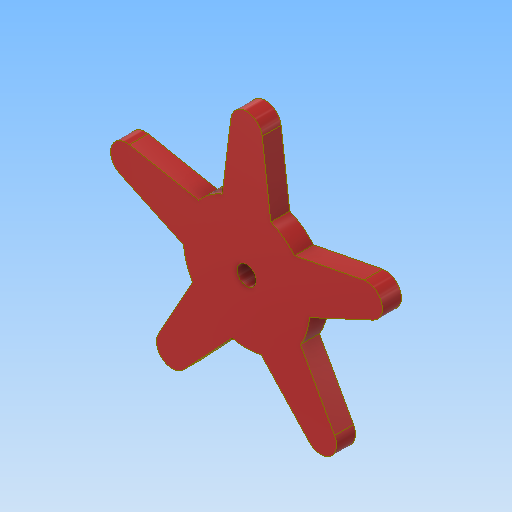
# Autodesk Inventor part: Selection_Gear 1
Saved by Autodesk Inventor 2018.1 (Build 221171000, 171)
## iProperties
Created: 2019-02-16
Part Number: Selection_Gear 1
Material: Nylon 6/6
Document SubType Name: Modeling
Designer: James
Density: 1.13 g/cm^3
Appearance: Nylon 6
Mass: 2.30103 g
Surface Area: 18.9934 cm^2
Volume: 2.03631 cm^3
Author: James
Autodesk Inventor part; units mm, degrees
ref_plane "YZ Plane" through (0, 0, 0) normal (1, 0, 0) x (0, 1, 0)
ref_plane "XZ Plane" through (0, 0, 0) normal (0, 1, 0) x (-1, 0, 0)
ref_plane "XY Plane" through (0, 0, 0) normal (0, 0, 1) x (1, 0, 0)
sketch "Sketch1" plane through (0, 0, 0) normal (0, 0, 1) x (1, 0, 0)
  circle A0 centre (0, 0) radius 10
  dimension "d0" = 20
  constraints: 1 centre point, 1 coincident
  measures "d0" diameter of A0
extrude "Extrusion1" add sketch "Sketch1" along normal blind 3
sketch "Sketch2" plane through (0, 0, 3) normal (0, 0, 1) x (1, 0, 0)
  point P0 (0, 0)
  point P1 (0, 0)
  constraints: 1 coincident
hole "Hole1" at (0, 0, 3) direction (0, 0, -1) diameter 3 end through all
sketch "Sketch4" plane through (0, 0, 3) normal (0, 0, 1) x (1, 0, 0)
  circle A0 centre (0, 0) radius 10 projected
  circle A1 centre (0, 20) radius 2.5
  circle A2 centre (0, 0) radius 1.5 projected
  circle A3 centre (0, 0) radius 4.9374
  line L0 (-4.9006, 0.6017) -> (-2.4814, 20.3047)
  line L1 (2.4814, 20.3047) -> (4.9006, 0.6017)
  dimension "d17" = 20
  dimension "d25" = 5
  dimension "d26" = 20
  dimension "d28" = 14
  constraints: 4 end point, 4 point on circle, 4 tangent, 2 centre point, 1 coincident, 1 vertical alignment
  measures "d17" diameter of A0
  measures "d25" diameter of A1
  measures "d26" distance of point (0, 0) A1.centre
  measures "d28" angle of L0 L1
extrude "Extrusion2" add sketch "Sketch4" against normal up to surface (3 mm away) contours L1 A3 L0 A0 | A0 L0 A1 L1 | A1 picked at (-0.6528, 8.2479)
pattern_circular "Circular Pattern1" count 5 over 360 about axis through (0, 0, -10) along (0, 0, 1) of "Extrusion2"
body "Solid1"
